Autodesk Fusion 360 part; units mm, degrees
(part 9 of 11)
  line L1964 (-0.0174, -45.4367) -> (0.0013, -45.4717)
  arc A128 (1.72, -193.2625) -> (1.3786, -193.1211) centre (1.52, -193.2625) ccw
  line L1965 (14.633, -219.988) -> (14.6722, -219.9945)
  arc A129 (1.72, -193.2625) -> (1.3786, -193.1211) centre (1.52, -193.2625) ccw
  line L1966 (14.6987, -220.198) -> (14.7482, -220.1997)
  line L1967 (6.02, -30.1995) -> (6.02, -32.839)
  line L1968 (3.3593, -195.4997) -> (1.72, -195.4997)
  line L1969 (3.7635, -37.4997) -> (7.1635, -34.0997)
  line L1970 (14.6722, -219.9945) -> (14.7117, -219.9984)
  line L1971 (6.02, -32.839) -> (3.3593, -35.4997)
  line L1972 (-0.0174, -45.4367) -> (0.0013, -45.4717)
  arc A130 (18.4614, -93.1211) -> (18.12, -93.2625) centre (18.32, -93.2625) ccw
  line L1973 (17.92, -144.6997) -> (17.92, -146.7368)
  line L1974 (19.9187, -145.2079) -> (19.92, -145.1682)
  line L1975 (15.42, -141.7997) -> (15.42, -143.439)
  arc A131 (18.4614, -93.1211) -> (18.12, -93.2625) centre (18.32, -93.2625) ccw
  line L1976 (17.92, -93.2625) -> (17.92, -95.2997)
  line L1977 (18.12, -93.2625) -> (18.12, -95.4997)
  line L1978 (16.4807, -144.4997) -> (18.12, -144.4997)
  line L1979 (16.4807, -144.4997) -> (18.12, -144.4997)
  line L1980 (18.12, -144.4997) -> (18.12, -146.7368)
  line L1981 (18.12, -93.2625) -> (18.12, -95.4997)
  line L1982 (19.7946, -94.4616) -> (19.7694, -94.4308)
  line L1983 (19.7422, -94.4019) -> (18.4614, -93.1211)
  line L1984 (16.5635, -144.6997) -> (17.92, -144.6997)
  arc A132 (18.12, -146.7368) -> (18.4614, -146.8782) centre (18.32, -146.7368) ccw
  arc A133 (18.6028, -92.9797) -> (17.92, -93.2625) centre (18.32, -93.2625) ccw
  line L1985 (19.7422, -94.4019) -> (18.4614, -93.1211)
  line L1986 (19.8859, -94.2627) -> (18.6028, -92.9797)
  arc A134 (18.12, -146.7368) -> (18.4614, -146.8782) centre (18.32, -146.7368) ccw
  line L1987 (14.7514, -139.9997) -> (18.42, -139.9997)
  line L1988 (15.42, -141.7997) -> (15.42, -143.439)
  arc A135 (17.92, -146.7368) -> (18.6028, -147.0197) centre (18.32, -146.7368) ccw
  line L1989 (18.42, -139.9997) -> (14.7514, -139.9997)
  line L1990 (19.92, -105.0997) -> (19.92, -94.8997)
  line L1991 (19.92, -105.0997) -> (19.92, -94.8997)
  line L1992 (19.7694, -94.4308) -> (19.7422, -94.4019)
  line L1993 (14.7482, -140.1997) -> (18.42, -140.1997)
  line L1994 (15.22, -141.9997) -> (15.22, -143.3562)
  line L1995 (19.7694, -94.4308) -> (19.7422, -94.4019)
  line L1996 (18.12, -144.4997) -> (18.12, -146.7368)
  line L1997 (20.12, -105.1009) -> (20.12, -94.8985)
  line L1998 (18.42, -139.9997) -> (14.7514, -139.9997)
  arc A136 (18.4614, -153.1211) -> (18.12, -153.2625) centre (18.32, -153.2625) ccw
  arc A137 (18.6028, -152.9797) -> (17.92, -153.2625) centre (18.32, -153.2625) ccw
  circle A138 centre (9.92, -149.9997) radius 2.1
  line L1999 (14.02, -152.7562) -> (14.02, -150.1167)
  line L2000 (16.1593, -157.2997) -> (18.12, -157.2997)
  line L2001 (17.92, -155.2997) -> (16.5635, -155.2997)
  line L2002 (18.12, -155.4997) -> (16.4807, -155.4997)
  arc A139 (18.4614, -153.1211) -> (18.12, -153.2625) centre (18.32, -153.2625) ccw
  line L2003 (18.12, -155.4997) -> (16.4807, -155.4997)
  line L2004 (10.127, -153.8997) -> (12.7593, -153.8997)
  line L2005 (13.82, -152.839) -> (13.82, -150.1995)
  line L2006 (5.82, -107.2432) -> (5.82, -109.8826)
  line L2007 (9.92, -153.6927) -> (10.127, -153.8997)
  line L2008 (13.903, -149.9997) -> (14.02, -149.8826)
  line L2009 (14.02, -150.1167) -> (13.903, -149.9997)
  circle A140 centre (9.92, -149.9997) radius 2.1
  line L2010 (9.92, -153.6927) -> (10.127, -153.8997)
  line L2011 (9.7959, -154.0997) -> (9.92, -153.9755)
  line L2012 (13.6201, -149.9997) -> (13.82, -149.7998)
  line L2013 (13.6201, -149.9997) -> (13.82, -149.7998)
  line L2014 (10.0441, -154.0997) -> (12.6765, -154.0997)
  line L2015 (14.3945, -80.1165) -> (14.4426, -80.1383)
  line L2016 (14.3222, -79.8219) -> (14.3512, -79.849)
  line L2017 (14.3819, -79.8742) -> (14.4142, -79.8974)
  line L2018 (16.5635, -124.6997) -> (17.92, -124.6997)
  line L2019 (14.483, -80.0623) -> (14.4479, -80.081)
  circle A141 centre (9.92, -129.9997) radius 2.1
  line L2020 (13.82, -130.1995) -> (13.6201, -129.9997)
  line L2021 (14.02, -132.7562) -> (14.02, -130.1167)
  line L2022 (14.4426, -79.861) -> (14.3945, -79.8828)
  line L2023 (14.3512, -79.849) -> (14.3819, -79.8742)
  line L2024 (14.3479, -79.9077) -> (14.303, -79.9356)
  line L2025 (14.4142, -80.102) -> (14.3819, -80.1251)
  line L2026 (14.483, -80.0623) -> (14.4479, -80.081)
  line L2027 (13.82, -130.1995) -> (13.6201, -129.9997)
  circle A142 centre (9.92, -129.9997) radius 2.1
  line L2028 (14.2601, -80.033) -> (14.303, -80.0637)
  line L2029 (14.5191, -80.0459) -> (14.483, -80.0623)
  line L2030 (14.3819, -79.8742) -> (14.4142, -79.8974)
  line L2031 (14.4142, -79.8974) -> (14.4479, -79.9183)
  line L2032 (14.3222, -79.8219) -> (14.3512, -79.849)
  line L2033 (14.7117, -79.9984) -> (14.7514, -79.9997)
  line L2034 (14.7117, -79.9984) -> (14.7514, -79.9997)
  line L2035 (1.72, -135.4997) -> (1.72, -133.2625)
  line L2036 (14.4426, -80.1383) -> (14.492, -80.1569)
  line L2037 (14.5425, -79.8271) -> (14.492, -79.8424)
  line L2038 (14.7514, -79.9997) -> (14.7117, -80.001)
  line L2039 (14.7482, -79.7997) -> (14.6987, -79.8013)
  line L2040 (6.02, -132.839) -> (3.3593, -135.4997)
  line L2041 (1.72, -135.4997) -> (1.72, -133.2625)
  line L2042 (14.5563, -80.0319) -> (14.5191, -80.0459)
  line L2043 (4.62, -136.6432) -> (7.1635, -134.0997)
  line L2044 (14.5563, -80.0319) -> (14.5191, -80.0459)
  line L2045 (3.2765, -135.2997) -> (1.92, -135.2997)
  line L2046 (14.5191, -79.9534) -> (14.5563, -79.9674)
  line L2047 (1.92, -135.2997) -> (1.92, -133.2625)
  line L2048 (14.6987, -80.198) -> (14.7482, -80.1997)
  arc A143 (1.72, -133.2625) -> (1.3786, -133.1211) centre (1.52, -133.2625) ccw
  line L2049 (14.3512, -80.1503) -> (14.3222, -80.1775)
  line L2050 (14.492, -80.1569) -> (14.5425, -80.1723)
  line L2051 (14.4479, -80.081) -> (14.4142, -80.102)
  line L2052 (14.5191, -79.9534) -> (14.5563, -79.9674)
  line L2053 (14.7514, -79.9997) -> (14.7117, -80.001)
  arc A144 (1.92, -133.2625) -> (1.2372, -132.9797) centre (1.52, -133.2625) ccw
  line L2054 (20.1184, -74.7783) -> (20.1132, -74.7258)
  line L2055 (19.8738, -74.5988) -> (19.8574, -74.5626)
  line L2056 (3.3593, -135.4997) -> (1.72, -135.4997)
  line L2057 (20.1046, -74.6736) -> (20.0926, -74.6222)
  line L2058 (6.02, -132.839) -> (3.3593, -135.4997)
  line L2059 (19.92, -74.8311) -> (19.9187, -74.7914)
  line L2060 (4.42, -136.5603) -> (7.0807, -133.8997)
  line L2061 (4.42, -136.5603) -> (7.0807, -133.8997)
  line L2062 (5.82, -132.7562) -> (3.2765, -135.2997)
  line L2063 (3.3593, -135.4997) -> (1.72, -135.4997)
  arc A145 (1.72, -133.2625) -> (1.3786, -133.1211) centre (1.52, -133.2625) ccw
  line L2064 (20.0926, -74.6222) -> (20.0773, -74.5717)
  line L2065 (20.1132, -74.7258) -> (20.1046, -74.6736)
  line L2066 (20.012, -74.4275) -> (19.9841, -74.3827)
  line L2067 (0.0978, -134.4019) -> (0.0706, -134.4308)
  line L2068 (19.8387, -74.5276) -> (19.8177, -74.4938)
  line L2069 (19.8387, -74.5276) -> (19.8177, -74.4938)
  line L2070 (19.9148, -74.7519) -> (19.9083, -74.7127)
  line L2071 (20.12, -78.4997) -> (20.12, -74.8278)
  line L2072 (-0.1969, -134.4741) -> (-0.2187, -134.5222)
  line L2073 (20.0773, -74.5717) -> (20.0587, -74.5222)
  line L2074 (19.9198, -74.2989) -> (19.8859, -74.2627)
  line L2075 (-0.2732, -134.7258) -> (-0.2786, -134.7804)
  line L2076 (19.8574, -74.5626) -> (19.8387, -74.5276)
  line L2077 (-0.172, -134.4275) -> (-0.1969, -134.4741)
  line L2078 (0.0454, -134.4616) -> (0.0223, -134.4938)
  line L2079 (20.12, -74.8278) -> (20.1184, -74.7783)
  line L2080 (-0.0174, -134.5626) -> (-0.0338, -134.5988)
  line L2081 (19.8993, -74.674) -> (19.8878, -74.636)
  line L2082 (-0.0478, -134.636) -> (-0.0593, -134.674)
  line L2083 (19.7694, -74.4308) -> (19.7422, -74.4019)
  line L2084 (19.8738, -74.5988) -> (19.8574, -74.5626)
  line L2085 (-0.0683, -134.7127) -> (-0.0748, -134.7519)
  line L2086 (-0.08, -54.8997) -> (-0.08, -65.0997)
  line L2087 (19.8177, -74.4938) -> (19.7946, -74.4616)
  line L2088 (0.0013, -134.5276) -> (-0.0174, -134.5626)
  line L2089 (-0.0593, -134.674) -> (-0.0683, -134.7127)
  line L2090 (-0.0683, -134.7127) -> (-0.0748, -134.7519)
  line L2091 (19.8878, -74.636) -> (19.8738, -74.5988)
  line L2092 (19.9187, -74.7914) -> (19.9148, -74.7519)
  line L2093 (-0.0787, -134.7914) -> (-0.08, -134.8997)
  line L2094 (-0.0338, -134.5988) -> (-0.0478, -134.636)
  line L2095 (-0.2187, -134.5222) -> (-0.2373, -134.5717)
  line L2096 (19.8177, -74.4938) -> (19.7946, -74.4616)
  line L2097 (20.0369, -74.4741) -> (20.012, -74.4275)
  line L2098 (19.8878, -74.636) -> (19.8738, -74.5988)
  line L2099 (-0.0748, -134.7519) -> (-0.0787, -134.7914)
  line L2100 (-0.0338, -134.5988) -> (-0.0478, -134.636)
  line L2101 (0.0978, -134.4019) -> (0.0706, -134.4308)
  line L2102 (19.9533, -74.3397) -> (19.9198, -74.2989)
  line L2103 (19.9841, -74.3827) -> (19.9533, -74.3397)
  line L2104 (19.7694, -74.4308) -> (19.7422, -74.4019)
  line L2105 (-0.0174, -134.5626) -> (-0.0338, -134.5988)
  line L2106 (19.9148, -74.7519) -> (19.9083, -74.7127)
  line L2107 (19.9187, -74.7914) -> (19.9148, -74.7519)
  line L2108 (-0.0478, -134.636) -> (-0.0593, -134.674)
  line L2109 (-0.1133, -134.3397) -> (-0.1441, -134.3827)
  line L2110 (19.8574, -74.5626) -> (19.8387, -74.5276)
  line L2111 (-0.2526, -134.6222) -> (-0.2646, -134.6736)
  line L2112 (19.9083, -74.7127) -> (19.8993, -74.674)
  line L2113 (0.0223, -134.4938) -> (0.0013, -134.5276)
  line L2114 (19.7946, -74.4616) -> (19.7694, -74.4308)
  line L2115 (-0.0798, -134.2989) -> (-0.1133, -134.3397)
  line L2116 (0.0706, -134.4308) -> (0.0454, -134.4616)
  line L2117 (1.92, -162.4997) -> (1.92, -157.4997)
  line L2118 (-0.0459, -134.2627) -> (-0.0798, -134.2989)
  line L2119 (17.92, -73.2625) -> (17.92, -75.2997)
  line L2120 (19.92, -74.8311) -> (19.9187, -74.7914)
  line L2121 (-0.2373, -134.5717) -> (-0.2526, -134.6222)
  line L2122 (-0.1441, -134.3827) -> (-0.172, -134.4275)
  line L2123 (-0.0787, -134.7914) -> (-0.08, -134.8997)
  line L2124 (20.0587, -74.5222) -> (20.0369, -74.4741)
  line L2125 (19.92, -78.4997) -> (19.92, -74.8311)
  line L2126 (0.0706, -134.4308) -> (0.0454, -134.4616)
  line L2127 (19.92, -78.4997) -> (19.92, -74.8311)
  line L2128 (-0.2646, -134.6736) -> (-0.2732, -134.7258)
  line L2129 (19.9083, -74.7127) -> (19.8993, -74.674)
  line L2130 (0.0013, -134.5276) -> (-0.0174, -134.5626)
  line L2131 (19.8993, -74.674) -> (19.8878, -74.636)
  line L2132 (19.7946, -74.4616) -> (19.7694, -74.4308)
  line L2133 (0.0223, -134.4938) -> (0.0013, -134.5276)
  line L2134 (-0.2786, -134.7804) -> (-0.28, -134.8985)
  line L2135 (18.12, -75.4997) -> (16.4807, -75.4997)
  line L2136 (5.937, -129.9997) -> (5.82, -130.1167)
  line L2137 (15.42, -76.5603) -> (15.42, -78.1997)
  arc A146 (18.4614, -73.1211) -> (18.12, -73.2625) centre (18.32, -73.2625) ccw
  line L2138 (1.3786, -133.1211) -> (0.0978, -134.4019)
  line L2139 (18.12, -73.2625) -> (18.12, -75.4997)
  line L2140 (1.2372, -132.9797) -> (-0.0459, -134.2627)
  line L2141 (19.8859, -74.2627) -> (18.6028, -72.9797)
  line L2142 (-0.0593, -134.674) -> (-0.0683, -134.7127)
  line L2143 (17.92, -75.2997) -> (16.5635, -75.2997)
  arc A147 (18.4614, -73.1211) -> (18.12, -73.2625) centre (18.32, -73.2625) ccw
  arc A148 (18.6028, -72.9797) -> (17.92, -73.2625) centre (18.32, -73.2625) ccw
  line L2144 (0.0454, -134.4616) -> (0.0223, -134.4938)
  line L2145 (15.22, -76.6432) -> (15.22, -77.9997)
  line L2146 (18.12, -73.2625) -> (18.12, -75.4997)
  line L2147 (-0.0748, -134.7519) -> (-0.0787, -134.7914)
  line L2148 (1.3786, -133.1211) -> (0.0978, -134.4019)
  line L2149 (15.42, -76.5603) -> (15.42, -78.1997)
  line L2150 (18.12, -75.4997) -> (16.4807, -75.4997)
  line L2151 (19.7422, -74.4019) -> (18.4614, -73.1211)
  arc A149 (1.3786, -126.8782) -> (1.72, -126.7368) centre (1.52, -126.7368) ccw
  line L2152 (19.7422, -74.4019) -> (18.4614, -73.1211)
  line L2153 (6.02, -127.1603) -> (6.02, -129.7998)
  line L2154 (19.92, -79.4997) -> (19.92, -78.4997)
  line L2155 (20.12, -79.4997) -> (20.12, -78.4997)
  line L2156 (5.82, -129.8826) -> (5.937, -129.9997)
  arc A150 (1.3786, -126.8782) -> (1.72, -126.7368) centre (1.52, -126.7368) ccw
  line L2157 (5.2837, -80.0319) -> (5.2457, -80.0203)
  line L2158 (19.9083, -114.7127) -> (19.8993, -114.674)
  line L2159 (19.8993, -114.674) -> (19.8878, -114.636)
  line L2160 (5.1678, -80.0049) -> (5.1283, -80.001)
  line L2161 (5.246, -79.8151) -> (5.1939, -79.8065)
  line L2162 (19.9148, -114.7519) -> (19.9083, -114.7127)
  line L2163 (18.12, -117.2997) -> (18.12, -122.6997)
  line L2164 (20.1046, -114.6736) -> (20.0926, -114.6222)
  line L2165 (19.8878, -114.636) -> (19.8738, -114.5988)
  line L2166 (5.1678, -79.9945) -> (5.207, -79.988)
  line L2167 (19.8878, -114.636) -> (19.8738, -114.5988)
  line L2168 (18.12, -122.6997) -> (16.1593, -122.6997)
  line L2169 (5.207, -80.0113) -> (5.1678, -80.0049)
  line L2170 (5.1678, -80.0049) -> (5.1283, -80.001)
  line L2171 (17.92, -122.4997) -> (16.0765, -122.4997)
  line L2172 (5.1283, -79.9984) -> (5.1678, -79.9945)
  line L2173 (19.9187, -114.7914) -> (19.9148, -114.7519)
  line L2174 (5.1413, -80.198) -> (5.1939, -80.1929)
  line L2175 (5.2457, -79.979) -> (5.2837, -79.9674)
  line L2176 (18.12, -117.2997) -> (18.12, -122.6997)
  line L2177 (5.2837, -80.0319) -> (5.2457, -80.0203)
  line L2178 (6.2199, -129.9997) -> (6.02, -130.1995)
  line L2179 (19.92, -65.0997) -> (19.92, -54.8997)
  arc A151 (1.2372, -127.0197) -> (1.92, -126.7368) centre (1.52, -126.7368) ccw
  line L2180 (12.9, -78.6825) -> (14.1831, -79.9656)
  line L2181 (10.0448, -74.0997) -> (12.6765, -74.0997)
  arc A152 (13.1828, -78.1997) -> (13.0414, -78.5411) centre (13.1828, -78.3997) ccw
  line L2182 (6.2199, -129.9997) -> (6.02, -130.1995)
  line L2183 (6.02, -129.7998) -> (6.2199, -129.9997)
  line L2184 (6.02, -129.7998) -> (6.2199, -129.9997)
  line L2185 (10.127, -73.8997) -> (12.7593, -73.8997)
  line L2186 (6.02, -127.1603) -> (6.02, -129.7998)
  line L2187 (9.7152, -73.8997) -> (9.92, -73.6949)
  arc A153 (13.1828, -77.9997) -> (12.9, -78.6825) centre (13.1828, -78.3997) ccw
  line L2188 (19.92, -79.4997) -> (19.92, -78.4997)
  line L2189 (9.7152, -73.8997) -> (9.92, -73.6949)
  line L2190 (10.127, -73.8997) -> (12.7593, -73.8997)
  line L2191 (9.7981, -74.0997) -> (9.9208, -73.977)
  line L2192 (9.92, -73.6949) -> (10.127, -73.8997)
  line L2193 (5.82, -127.2432) -> (5.82, -129.8826)
  line L2194 (1.72, -62.6997) -> (1.72, -57.2997)
  line L2195 (1.72, -124.4997) -> (3.3593, -124.4997)
  line L2196 (-0.2373, -125.4277) -> (-0.2187, -125.4771)
  line L2197 (9.92, -73.6949) -> (10.127, -73.8997)
  line L2198 (12.6765, -74.0997) -> (15.22, -76.6432)
  line L2199 (-0.2526, -125.3771) -> (-0.2373, -125.4277)
  arc A154 (13.1828, -78.1997) -> (13.0414, -78.5411) centre (13.1828, -78.3997) ccw
  line L2200 (-0.0748, -125.2474) -> (-0.0683, -125.2866)
  line L2201 (16.5635, -75.2997) -> (14.02, -72.7562)
  line L2202 (9.9208, -73.977) -> (10.0448, -74.0997)
  line L2203 (12.7593, -73.8997) -> (15.42, -76.5603)
  line L2204 (0.0013, -125.4717) -> (0.0223, -125.5055)
  line L2205 (13.0414, -78.5411) -> (14.3222, -79.8219)
  line L2206 (-0.28, -125.1009) -> (-0.2786, -125.2189)
  line L2207 (-0.1133, -125.6596) -> (-0.0798, -125.7004)
  line L2208 (-0.08, -125.0997) -> (-0.0787, -125.2079)
  line L2209 (15.42, -78.1997) -> (13.1828, -78.1997)
  line L2210 (0.0706, -125.5685) -> (0.0978, -125.5975)
  line L2211 (16.4807, -75.4997) -> (13.82, -72.839)
  line L2212 (14.1831, -79.9656) -> (14.2193, -79.9995)
  line L2213 (-0.0478, -125.3633) -> (-0.0338, -125.4005)
  line L2214 (15.42, -78.1997) -> (13.1828, -78.1997)
  line L2215 (12.7593, -73.8997) -> (15.42, -76.5603)
  line L2216 (-0.0593, -125.3253) -> (-0.0478, -125.3633)
  line L2217 (15.22, -77.9997) -> (13.1828, -77.9997)
  line L2218 (-0.0683, -125.2866) -> (-0.0593, -125.3253)
  line L2219 (13.0414, -78.5411) -> (14.3222, -79.8219)
  line L2220 (14.2193, -79.9999) -> (14.1831, -80.0337)
  line L2221 (-0.1441, -125.6166) -> (-0.1133, -125.6596)
  line L2222 (-0.0787, -125.2079) -> (-0.0748, -125.2474)
  line L2223 (-0.2786, -125.2189) -> (-0.2732, -125.2736)
  line L2224 (5.6569, -80.0337) -> (5.6207, -79.9999)
  line L2225 (-0.0338, -125.4005) -> (-0.0174, -125.4367)
  line L2226 (-0.2187, -125.4771) -> (-0.1969, -125.5252)
  line L2227 (-0.0787, -125.2079) -> (-0.0748, -125.2474)
  line L2228 (1.92, -124.6997) -> (3.2765, -124.6997)
  line L2229 (-0.0478, -125.3633) -> (-0.0338, -125.4005)
  line L2230 (5.6207, -79.9999) -> (5.5799, -79.9663)
  line L2231 (0.0454, -125.5378) -> (0.0706, -125.5685)
  line L2232 (-0.172, -125.5718) -> (-0.1441, -125.6166)
  line L2233 (-0.2646, -125.3257) -> (-0.2526, -125.3771)
  line L2234 (16.4807, -75.4997) -> (13.82, -72.839)
  line L2235 (5.537, -80.0637) -> (5.5799, -80.033)
  line L2236 (-0.08, -125.0997) -> (-0.0787, -125.2079)
  line L2237 (-0.0174, -125.4367) -> (0.0013, -125.4717)
  line L2238 (5.5799, -79.9663) -> (5.537, -79.9356)
  line L2239 (-0.0593, -125.3253) -> (-0.0478, -125.3633)
  line L2240 (-0.0174, -125.4367) -> (0.0013, -125.4717)
  line L2241 (0.0223, -125.5055) -> (0.0454, -125.5378)
  line L2242 (5.6207, -79.9995) -> (5.6569, -79.9656)
  line L2243 (0.0454, -125.5378) -> (0.0706, -125.5685)
  line L2244 (-0.1969, -125.5252) -> (-0.172, -125.5718)
  line L2245 (0.0013, -125.4717) -> (0.0223, -125.5055)
  line L2246 (-0.0748, -125.2474) -> (-0.0683, -125.2866)
  line L2247 (1.72, -124.4997) -> (3.3593, -124.4997)
  line L2248 (5.4581, -80.1251) -> (5.4258, -80.102)
  line L2249 (-0.2732, -125.2736) -> (-0.2646, -125.3257)
  line L2250 (0.0223, -125.5055) -> (0.0454, -125.5378)
  line L2251 (0.0706, -125.5685) -> (0.0978, -125.5975)
  line L2252 (-0.0798, -125.7004) -> (-0.0459, -125.7366)
  line L2253 (-0.0683, -125.2866) -> (-0.0593, -125.3253)
  line L2254 (5.3921, -80.081) -> (5.357, -80.0623)
  line L2255 (5.5799, -80.033) -> (5.6207, -79.9995)
  line L2256 (-0.0338, -125.4005) -> (-0.0174, -125.4367)
  line L2257 (5.4258, -79.8974) -> (5.4581, -79.8742)
  line L2258 (5.348, -80.1569) -> (5.3974, -80.1383)
  line L2259 (-0.0459, -125.7366) -> (1.2372, -127.0197)
  line L2260 (0.0978, -125.5975) -> (1.3786, -126.8782)
  line L2261 (5.4581, -79.8742) -> (5.4888, -79.849)
  line L2262 (5.357, -80.0623) -> (5.3209, -80.0459)
  line L2263 (6.02, -130.1995) -> (6.02, -132.839)
  line L2264 (1.72, -126.7368) -> (1.72, -124.4997)
  line L2265 (5.3974, -79.861) -> (5.348, -79.8424)
  line L2266 (5.4455, -79.8828) -> (5.3974, -79.861)
  line L2267 (1.92, -126.7368) -> (1.92, -124.6997)
  line L2268 (5.357, -79.9371) -> (5.3921, -79.9183)
  line L2269 (5.4455, -80.1165) -> (5.4921, -80.0916)
  line L2270 (0.0978, -125.5975) -> (1.3786, -126.8782)
  line L2271 (1.72, -126.7368) -> (1.72, -124.4997)
  line L2272 (5.4888, -80.1503) -> (5.4581, -80.1251)
  line L2273 (3.3593, -124.4997) -> (6.02, -127.1603)
  line L2274 (5.3921, -79.9183) -> (5.4258, -79.8974)
  line L2275 (3.3593, -124.4997) -> (6.02, -127.1603)
  line L2276 (3.2765, -124.6997) -> (5.82, -127.2432)
  line L2277 (5.82, -130.1167) -> (5.82, -132.7562)
  line L2278 (5.4258, -80.102) -> (5.3921, -80.081)
  line L2279 (5.3921, -79.9183) -> (5.4258, -79.8974)
  line L2280 (5.357, -79.9371) -> (5.3921, -79.9183)
  line L2281 (5.1939, -79.8065) -> (5.1413, -79.8013)
  line L2282 (7.0807, -133.8997) -> (9.7152, -133.8997)
  line L2283 (5.207, -79.988) -> (5.2457, -79.979)
  line L2284 (5.4258, -79.8974) -> (5.4581, -79.8742)
  line L2285 (5.3209, -79.9534) -> (5.357, -79.9371)
  line L2286 (7.1635, -134.0997) -> (9.7981, -134.0997)
  line L2287 (5.3921, -80.081) -> (5.357, -80.0623)
  line L2288 (5.4921, -79.9077) -> (5.4455, -79.8828)
  line L2289 (5.3209, -79.9534) -> (5.357, -79.9371)
  line L2290 (5.4888, -80.1503) -> (5.4581, -80.1251)
  line L2291 (7.0807, -133.8997) -> (9.7152, -133.8997)
  line L2292 (9.7959, -125.8997) -> (7.1635, -125.8997)
  line L2293 (5.357, -80.0623) -> (5.3209, -80.0459)
  line L2294 (9.713, -126.0997) -> (7.0807, -126.0997)
  line L2295 (5.4581, -80.1251) -> (5.4258, -80.102)
  line L2296 (9.713, -126.0997) -> (7.0807, -126.0997)
  line L2297 (6.02, -130.1995) -> (6.02, -132.839)
  line L2298 (5.3974, -80.1383) -> (5.4455, -80.1165)
  line L2299 (5.4581, -79.8742) -> (5.4888, -79.849)
  line L2300 (5.4258, -80.102) -> (5.3921, -80.081)
  line L2301 (5.1283, -79.9984) -> (5.1678, -79.9945)
  line L2302 (19.9187, -114.7914) -> (19.9148, -114.7519)
  line L2303 (5.2457, -80.0203) -> (5.207, -80.0113)
  line L2304 (0.0706, -154.4308) -> (0.0454, -154.4616)
  arc A155 (1.72, -153.2625) -> (1.3786, -153.1211) centre (1.52, -153.2625) ccw
  line L2305 (19.9083, -105.2866) -> (19.9148, -105.2474)
  line L2306 (6.2199, -149.9997) -> (6.02, -150.1995)
  line L2307 (-0.2526, -154.6222) -> (-0.2646, -154.6736)
  line L2308 (-0.0174, -154.5626) -> (-0.0338, -154.5988)
  line L2309 (0.0223, -154.4938) -> (0.0013, -154.5276)
  line L2310 (20.1186, -105.2189) -> (20.12, -105.1009)
  line L2311 (0.0223, -154.4938) -> (0.0013, -154.5276)
  line L2312 (-0.1441, -154.3827) -> (-0.172, -154.4275)
  line L2313 (0.0978, -154.4019) -> (0.0706, -154.4308)
  line L2314 (-0.172, -154.4275) -> (-0.1969, -154.4741)
  line L2315 (-0.0787, -154.7914) -> (-0.08, -154.8997)
  line L2316 (0.0706, -154.4308) -> (0.0454, -154.4616)
  arc A156 (1.92, -153.2625) -> (1.2372, -152.9797) centre (1.52, -153.2625) ccw
  line L2317 (-0.0478, -154.636) -> (-0.0593, -154.674)
  line L2318 (19.9841, -105.6166) -> (20.012, -105.5718)
  arc A157 (1.72, -153.2625) -> (1.3786, -153.1211) centre (1.52, -153.2625) ccw
  line L2319 (19.8177, -105.5055) -> (19.8387, -105.4717)
  line L2320 (20.1046, -105.3257) -> (20.1132, -105.2736)
  line L2321 (19.7946, -105.5378) -> (19.8177, -105.5055)
  line L2322 (19.8387, -105.4717) -> (19.8574, -105.4367)
  line L2323 (6.02, -152.839) -> (3.3593, -155.4997)
  line L2324 (19.9148, -105.2474) -> (19.9187, -105.2079)
  line L2325 (19.9187, -105.2079) -> (19.92, -105.0997)
  line L2326 (19.9148, -105.2474) -> (19.9187, -105.2079)
  line L2327 (19.9198, -105.7004) -> (19.9533, -105.6596)
  line L2328 (6.2199, -149.9997) -> (6.02, -150.1995)
  line L2329 (5.82, -149.8826) -> (5.937, -149.9997)
  line L2330 (20.0587, -105.4771) -> (20.0773, -105.4277)
  line L2331 (5.937, -149.9997) -> (5.82, -150.1167)
  line L2332 (6.02, -150.1995) -> (6.02, -152.839)
  line L2333 (6.02, -149.7998) -> (6.2199, -149.9997)
  line L2334 (5.82, -150.1167) -> (5.82, -152.7562)
  line L2335 (6.02, -150.1995) -> (6.02, -152.839)
  line L2336 (19.8574, -105.4367) -> (19.8738, -105.4005)
  line L2337 (6.02, -149.7998) -> (6.2199, -149.9997)
  line L2338 (19.8878, -105.3633) -> (19.8993, -105.3253)
  line L2339 (19.9533, -105.6596) -> (19.9841, -105.6166)
  line L2340 (1.72, -155.4997) -> (1.72, -153.2625)
  line L2341 (19.8878, -105.3633) -> (19.8993, -105.3253)
  line L2342 (20.012, -105.5718) -> (20.0369, -105.5252)
  line L2343 (20.1186, -94.7804) -> (20.1132, -94.7258)
  line L2344 (20.0369, -94.4741) -> (20.012, -94.4275)
  line L2345 (19.7694, -145.5685) -> (19.7946, -145.5378)
  line L2346 (19.8993, -145.3253) -> (19.9083, -145.2866)
  line L2347 (19.8878, -94.636) -> (19.8738, -94.5988)
  line L2348 (19.9148, -145.2474) -> (19.9187, -145.2079)
  line L2349 (20.0926, -94.6222) -> (20.0773, -94.5717)
  line L2350 (19.9841, -145.6166) -> (20.012, -145.5718)
  line L2351 (19.7946, -145.5378) -> (19.8177, -145.5055)
  line L2352 (20.12, -94.8985) -> (20.1186, -94.7804)
  line L2353 (19.8177, -94.4938) -> (19.7946, -94.4616)
  line L2354 (19.8738, -145.4005) -> (19.8878, -145.3633)
  line L2355 (20.1132, -145.2736) -> (20.1184, -145.221)
  line L2356 (20.0926, -145.3771) -> (20.1046, -145.3257)
  line L2357 (19.9198, -145.7004) -> (19.9533, -145.6596)
  line L2358 (19.8993, -94.674) -> (19.8878, -94.636)
  line L2359 (19.9198, -94.2989) -> (19.8859, -94.2627)
  line L2360 (19.8177, -145.5055) -> (19.8387, -145.4717)
  line L2361 (19.8574, -94.5626) -> (19.8387, -94.5276)
  line L2362 (20.012, -94.4275) -> (19.9841, -94.3827)
  line L2363 (20.1046, -145.3257) -> (20.1132, -145.2736)
  line L2364 (19.8859, -145.7366) -> (19.9198, -145.7004)
  line L2365 (17.92, -97.4997) -> (17.92, -102.4997)
  line L2366 (19.8387, -145.4717) -> (19.8574, -145.4367)
  line L2367 (19.7946, -145.5378) -> (19.8177, -145.5055)
  line L2368 (19.8177, -145.5055) -> (19.8387, -145.4717)
  line L2369 (18.6028, -107.0197) -> (19.8859, -105.7366)
  line L2370 (18.12, -97.2997) -> (18.12, -102.6997)
  line L2371 (18.12, -97.2997) -> (18.12, -102.6997)
  line L2372 (20.0773, -145.4277) -> (20.0926, -145.3771)
  line L2373 (19.8387, -145.4717) -> (19.8574, -145.4367)
  line L2374 (19.9148, -145.2474) -> (19.9187, -145.2079)
  line L2375 (19.9533, -145.6596) -> (19.9841, -145.6166)
  line L2376 (19.7422, -145.5975) -> (19.7694, -145.5685)
  line L2377 (20.0587, -145.4771) -> (20.0773, -145.4277)
  line L2378 (20.012, -145.5718) -> (20.0369, -145.5252)
  line L2379 (-0.2187, -154.5222) -> (-0.2373, -154.5717)
  line L2380 (0.0013, -154.5276) -> (-0.0174, -154.5626)
  line L2381 (-0.2646, -154.6736) -> (-0.2732, -154.7258)
  line L2382 (-0.0748, -154.7519) -> (-0.0787, -154.7914)
  line L2383 (-0.0593, -154.674) -> (-0.0683, -154.7127)
  line L2384 (-0.0338, -154.5988) -> (-0.0478, -154.636)
  line L2385 (-0.0787, -154.7914) -> (-0.08, -154.8997)
  line L2386 (-0.0174, -154.5626) -> (-0.0338, -154.5988)
  line L2387 (0.0013, -154.5276) -> (-0.0174, -154.5626)
  line L2388 (-0.0593, -154.674) -> (-0.0683, -154.7127)
  line L2389 (-0.0338, -154.5988) -> (-0.0478, -154.636)
  line L2390 (-0.0748, -154.7519) -> (-0.0787, -154.7914)
  line L2391 (-0.1133, -154.3397) -> (-0.1441, -154.3827)
  line L2392 (-0.0798, -154.2989) -> (-0.1133, -154.3397)
  line L2393 (0.0454, -154.4616) -> (0.0223, -154.4938)
  line L2394 (-0.1969, -154.4741) -> (-0.2187, -154.5222)
  line L2395 (-0.0459, -154.2627) -> (-0.0798, -154.2989)
  line L2396 (-0.2373, -154.5717) -> (-0.2526, -154.6222)
  line L2397 (-0.0478, -154.636) -> (-0.0593, -154.674)
  line L2398 (0.0978, -154.4019) -> (0.0706, -154.4308)
  line L2399 (-0.2786, -154.7804) -> (-0.28, -154.8985)
  line L2400 (-0.0683, -154.7127) -> (-0.0748, -154.7519)
  line L2401 (-0.2732, -154.7258) -> (-0.2786, -154.7804)
  line L2402 (-0.0683, -154.7127) -> (-0.0748, -154.7519)
  line L2403 (19.9148, -154.7519) -> (19.9083, -154.7127)
  line L2404 (20.0587, -154.5222) -> (20.0369, -154.4741)
  line L2405 (19.7694, -154.4308) -> (19.7422, -154.4019)
  line L2406 (20.1132, -154.7258) -> (20.1046, -154.6736)
  line L2407 (3.3593, -115.4997) -> (1.72, -115.4997)
  line L2408 (-0.2646, -114.6736) -> (-0.2732, -114.7258)
  line L2409 (-0.0593, -114.674) -> (-0.0683, -114.7127)
  line L2410 (-0.0478, -74.636) -> (-0.0593, -74.674)
  line L2411 (0.0706, -74.4308) -> (0.0454, -74.4616)
  line L2412 (-0.0478, -74.636) -> (-0.0593, -74.674)
  line L2413 (-0.0748, -74.7519) -> (-0.0787, -74.7914)
  line L2414 (3.6807, -122.6997) -> (1.72, -122.6997)
  line L2415 (0.0013, -114.5276) -> (-0.0174, -114.5626)
  line L2416 (-0.0593, -114.674) -> (-0.0683, -114.7127)
  line L2417 (-0.0174, -114.5626) -> (-0.0338, -114.5988)
  line L2418 (-0.0748, -74.7519) -> (-0.0787, -74.7914)
  line L2419 (1.72, -122.6997) -> (1.72, -117.2997)
  line L2420 (1.72, -122.6997) -> (1.72, -117.2997)
  line L2421 (-0.0338, -74.5988) -> (-0.0478, -74.636)
  line L2422 (0.0223, -74.4938) -> (0.0013, -74.5276)
  line L2423 (1.72, -117.2997) -> (3.6807, -117.2997)
  line L2424 (0.0454, -74.4616) -> (0.0223, -74.4938)
  line L2425 (-0.2786, -114.7804) -> (-0.28, -114.8985)
  line L2426 (-0.0683, -114.7127) -> (-0.0748, -114.7519)
  line L2427 (0.0223, -74.4938) -> (0.0013, -74.5276)
  line L2428 (-0.2373, -74.5717) -> (-0.2526, -74.6222)
  line L2429 (-0.0787, -114.7914) -> (-0.08, -114.8997)
  line L2430 (-0.2732, -114.7258) -> (-0.2786, -114.7804)
  line L2431 (-0.2646, -74.6736) -> (-0.2732, -74.7258)
  line L2432 (-0.0338, -114.5988) -> (-0.0478, -114.636)
  line L2433 (-0.28, -74.8985) -> (-0.28, -78.4997)
  line L2434 (-0.0787, -114.7914) -> (-0.08, -114.8997)
  line L2435 (-0.0683, -74.7127) -> (-0.0748, -74.7519)
  line L2436 (18.12, -157.2997) -> (18.12, -162.6997)
  line L2437 (0.0978, -74.4019) -> (0.0706, -74.4308)
  line L2438 (-0.0748, -114.7519) -> (-0.0787, -114.7914)
  line L2439 (-0.08, -74.8997) -> (-0.08, -78.4997)
  line L2440 (-0.2373, -114.5717) -> (-0.2526, -114.6222)
  line L2441 (-0.2187, -114.5222) -> (-0.2373, -114.5717)
  line L2442 (0.0013, -74.5276) -> (-0.0174, -74.5626)
  line L2443 (0.0013, -74.5276) -> (-0.0174, -74.5626)
  line L2444 (3.3593, -115.4997) -> (1.72, -115.4997)
  line L2445 (-0.1441, -74.3827) -> (-0.172, -74.4275)
  line L2446 (-0.2526, -74.6222) -> (-0.2646, -74.6736)
  line L2447 (1.92, -117.4997) -> (3.7635, -117.4997)
  line L2448 (-0.0683, -114.7127) -> (-0.0748, -114.7519)
  line L2449 (-0.1969, -74.4741) -> (-0.2187, -74.5222)
  line L2450 (1.72, -117.2997) -> (3.6807, -117.2997)
  line L2451 (0.0706, -74.4308) -> (0.0454, -74.4616)
  line L2452 (-0.0787, -74.7914) -> (-0.08, -74.8997)
  line L2453 (3.7635, -122.4997) -> (1.92, -122.4997)
  line L2454 (3.2765, -115.2997) -> (1.92, -115.2997)
  line L2455 (3.6807, -122.6997) -> (1.72, -122.6997)
  line L2456 (-0.0174, -74.5626) -> (-0.0338, -74.5988)
  line L2457 (0.0978, -74.4019) -> (0.0706, -74.4308)
  line L2458 (1.3786, -113.1211) -> (0.0978, -114.4019)
  line L2459 (1.2372, -72.9797) -> (-0.0459, -74.2627)
  line L2460 (-0.172, -74.4275) -> (-0.1969, -74.4741)
  arc A158 (1.92, -113.2625) -> (1.2372, -112.9797) centre (1.52, -113.2625) ccw
  line L2461 (1.3786, -73.1211) -> (0.0978, -74.4019)
  line L2462 (-0.0459, -74.2627) -> (-0.0798, -74.2989)
  line L2463 (-0.0338, -74.5988) -> (-0.0478, -74.636)
  line L2464 (-0.0174, -114.5626) -> (-0.0338, -114.5988)
  line L2465 (-0.0174, -74.5626) -> (-0.0338, -74.5988)
  arc A159 (1.72, -113.2625) -> (1.3786, -113.1211) centre (1.52, -113.2625) ccw
  line L2466 (-0.0593, -74.674) -> (-0.0683, -74.7127)
  line L2467 (-0.08, -74.8997) -> (-0.08, -78.4997)
  line L2468 (0.0013, -114.5276) -> (-0.0174, -114.5626)
  line L2469 (-0.2526, -114.6222) -> (-0.2646, -114.6736)
  line L2470 (-0.0787, -74.7914) -> (-0.08, -74.8997)
  line L2471 (-0.0748, -114.7519) -> (-0.0787, -114.7914)
  line L2472 (-0.2187, -74.5222) -> (-0.2373, -74.5717)
  line L2473 (-0.0338, -114.5988) -> (-0.0478, -114.636)
  line L2474 (-0.0683, -74.7127) -> (-0.0748, -74.7519)
  line L2475 (-0.1133, -74.3397) -> (-0.1441, -74.3827)
  line L2476 (0.0454, -74.4616) -> (0.0223, -74.4938)
  line L2477 (-0.0593, -74.674) -> (-0.0683, -74.7127)
  line L2478 (-0.172, -114.4275) -> (-0.1969, -114.4741)
  line L2479 (-0.0798, -114.2989) -> (-0.1133, -114.3397)
  arc A160 (1.72, -113.2625) -> (1.3786, -113.1211) centre (1.52, -113.2625) ccw
  line L2480 (0.0978, -114.4019) -> (0.0706, -114.4308)
  line L2481 (0.0706, -114.4308) -> (0.0454, -114.4616)
  line L2482 (5.6569, -79.9656) -> (6.94, -78.6825)
  line L2483 (1.3786, -73.1211) -> (0.0978, -74.4019)
  line L2484 (0.0706, -114.4308) -> (0.0454, -114.4616)
  line L2485 (-0.08, -78.4997) -> (-0.08, -79.4997)
  line L2486 (5.5178, -79.8219) -> (6.7986, -78.5411)
  line L2487 (0.0978, -114.4019) -> (0.0706, -114.4308)
  line L2488 (7.1635, -74.0997) -> (9.7981, -74.0997)
  line L2489 (-0.08, -78.4997) -> (-0.08, -79.4997)
  line L2490 (-0.28, -78.4997) -> (-0.28, -79.4997)
  line L2491 (-0.1441, -114.3827) -> (-0.172, -114.4275)
  line L2492 (7.0807, -73.8997) -> (9.7152, -73.8997)
  line L2493 (-0.0459, -114.2627) -> (-0.0798, -114.2989)
  line L2494 (1.2372, -112.9797) -> (-0.0459, -114.2627)
  line L2495 (5.5178, -79.8219) -> (6.7986, -78.5411)
  line L2496 (7.0807, -73.8997) -> (9.7152, -73.8997)
  line L2497 (1.3786, -113.1211) -> (0.0978, -114.4019)
  line L2498 (-0.1133, -114.3397) -> (-0.1441, -114.3827)
  line L2499 (0.0454, -114.4616) -> (0.0223, -114.4938)
  line L2500 (5.82, -112.7562) -> (3.2765, -115.2997)
  line L2501 (13.82, -70.1995) -> (13.6201, -69.9997)
  line L2502 (-0.1969, -114.4741) -> (-0.2187, -114.5222)
  line L2503 (6.02, -109.7998) -> (6.2199, -109.9997)
  line L2504 (0.0454, -114.4616) -> (0.0223, -114.4938)
  line L2505 (13.903, -69.9997) -> (14.02, -69.8826)
  line L2506 (6.02, -109.7998) -> (6.2199, -109.9997)
  line L2507 (6.02, -110.1995) -> (6.02, -112.839)
  line L2508 (14.02, -69.8826) -> (14.02, -67.2432)
  line L2509 (6.2199, -109.9997) -> (6.02, -110.1995)
  arc A161 (18.12, -66.7368) -> (18.4614, -66.8782) centre (18.32, -66.7368) ccw
  line L2510 (3.7635, -117.4997) -> (7.1635, -114.0997)
  line L2511 (13.82, -69.7998) -> (13.82, -67.1603)
  line L2512 (5.82, -110.1167) -> (5.82, -112.7562)
  line L2513 (5.82, -109.8826) -> (5.937, -109.9997)
  line L2514 (6.02, -110.1995) -> (6.02, -112.839)
  arc A162 (17.92, -66.7368) -> (18.6028, -67.0197) centre (18.32, -66.7368) ccw
  arc A163 (18.12, -66.7368) -> (18.4614, -66.8782) centre (18.32, -66.7368) ccw
  line L2515 (6.2199, -109.9997) -> (6.02, -110.1995)
  line L2516 (5.937, -109.9997) -> (5.82, -110.1167)
  line L2517 (14.02, -70.1167) -> (13.903, -69.9997)
  line L2518 (0.0223, -114.4938) -> (0.0013, -114.5276)
  line L2519 (7.0807, -113.8997) -> (9.713, -113.8997)
  line L2520 (16.0765, -122.4997) -> (12.6765, -125.8997)
  line L2521 (3.6807, -117.2997) -> (7.0807, -113.8997)
  line L2522 (7.0807, -113.8997) -> (9.713, -113.8997)
  line L2523 (6.02, -112.839) -> (3.3593, -115.4997)
  line L2524 (0.0223, -114.4938) -> (0.0013, -114.5276)
  line L2525 (13.82, -69.7998) -> (13.82, -67.1603)
  line L2526 (7.1635, -114.0997) -> (9.7959, -114.0997)
  line L2527 (6.02, -112.839) -> (3.3593, -115.4997)
  line L2528 (3.6807, -117.2997) -> (7.0807, -113.8997)
  line L2529 (13.82, -70.1995) -> (13.6201, -69.9997)
  line L2530 (1.92, -115.2997) -> (1.92, -113.2625)
  line L2531 (13.6201, -69.9997) -> (13.82, -69.7998)
  line L2532 (13.6201, -69.9997) -> (13.82, -69.7998)
  line L2533 (1.72, -115.4997) -> (1.72, -113.2625)
  line L2534 (1.72, -115.4997) -> (1.72, -113.2625)
  line L2535 (4.42, -138.1997) -> (4.42, -136.5603)
  line L2536 (19.8993, -65.3253) -> (19.9083, -65.2866)
  line L2537 (-0.08, -114.8997) -> (-0.08, -125.0997)
  line L2538 (7.1635, -125.8997) -> (3.7635, -122.4997)
  line L2539 (20.0773, -65.4277) -> (20.0926, -65.3771)
  line L2540 (19.92, -125.0997) -> (19.92, -114.8997)
  line L2541 (20.1132, -65.2736) -> (20.1186, -65.2189)
  line L2542 (19.92, -125.0997) -> (19.92, -114.8997)
  line L2543 (20.0926, -65.3771) -> (20.1046, -65.3257)
  line L2544 (16.1593, -122.6997) -> (12.7593, -126.0997)
  line L2545 (-0.08, -114.8997) -> (-0.08, -125.0997)
  line L2546 (20.12, -125.1009) -> (20.12, -114.8985)
  line L2547 (-0.28, -114.8985) -> (-0.28, -125.1009)
  line L2548 (7.0807, -126.0997) -> (3.6807, -122.6997)
  line L2549 (19.9187, -65.2079) -> (19.92, -65.0997)
  line L2550 (19.8177, -65.5055) -> (19.8387, -65.4717)
  line L2551 (20.1186, -65.2189) -> (20.12, -65.1009)
  line L2552 (19.8738, -65.4005) -> (19.8878, -65.3633)
  line L2553 (16.1593, -122.6997) -> (12.7593, -126.0997)
  line L2554 (-0.08, -134.8997) -> (-0.08, -138.4997)
  line L2555 (7.0807, -126.0997) -> (3.6807, -122.6997)
  line L2556 (19.9083, -65.2866) -> (19.9148, -65.2474)
  line L2557 (19.8387, -65.4717) -> (19.8574, -65.4367)
  line L2558 (19.9533, -65.6596) -> (19.9841, -65.6166)
  line L2559 (19.92, -138.4997) -> (19.92, -134.8311)
  line L2560 (19.7946, -65.5378) -> (19.8177, -65.5055)
  line L2561 (-0.28, -134.8985) -> (-0.28, -138.4997)
  line L2562 (15.42, -136.5603) -> (15.42, -138.1997)
  line L2563 (5.82, -192.7562) -> (3.2765, -195.2997)
  line L2564 (-0.0798, -205.7004) -> (-0.0459, -205.7366)
  line L2565 (5.4581, -219.8742) -> (5.4888, -219.849)
  line L2566 (6.2199, -189.9997) -> (6.02, -190.1995)
  line L2567 (0.0978, -165.5975) -> (1.3786, -166.8782)
  line L2568 (-0.2373, -165.4277) -> (-0.2187, -165.4771)
  line L2569 (-0.0174, -205.4367) -> (0.0013, -205.4717)
  line L2570 (5.3974, -220.1383) -> (5.4455, -220.1165)
  arc A164 (1.3786, -186.8782) -> (1.72, -186.7368) centre (1.52, -186.7368) ccw
  line L2571 (-0.1969, -205.5252) -> (-0.172, -205.5718)
  line L2572 (6.02, -189.7998) -> (6.2199, -189.9997)
  line L2573 (-0.1969, -165.5252) -> (-0.172, -165.5718)
  line L2574 (5.937, -189.9997) -> (5.82, -190.1167)
  line L2575 (-0.08, -205.0997) -> (-0.0787, -205.2079)
  line L2576 (-0.1441, -205.6166) -> (-0.1133, -205.6596)
  line L2577 (5.4921, -220.0916) -> (5.537, -220.0637)
  line L2578 (-0.0478, -205.3633) -> (-0.0338, -205.4005)
  line L2579 (-0.2786, -165.2189) -> (-0.2732, -165.2736)
  line L2580 (-0.2732, -165.2736) -> (-0.2646, -165.3257)
  line L2581 (5.0886, -219.9997) -> (5.1283, -219.9984)
  line L2582 (7.0807, -206.0997) -> (3.6807, -202.6997)
  line L2583 (-0.08, -194.8997) -> (-0.08, -205.0997)
  line L2584 (1.42, -220.1997) -> (5.0918, -220.1997)
  line L2585 (-0.2187, -205.4771) -> (-0.1969, -205.5252)
  line L2586 (0.0013, -205.4717) -> (0.0223, -205.5055)
  line L2587 (6.02, -167.1603) -> (6.02, -169.7998)
  line L2588 (5.1678, -219.9945) -> (5.207, -219.988)
  line L2589 (-0.0787, -205.2079) -> (-0.0748, -205.2474)
  line L2590 (1.42, -219.9997) -> (5.0886, -219.9997)
  line L2591 (5.82, -189.8826) -> (5.937, -189.9997)
  line L2592 (6.02, -187.1603) -> (6.02, -189.7998)
  line L2593 (5.4258, -219.8974) -> (5.4581, -219.8742)
  line L2594 (-0.28, -205.1009) -> (-0.2786, -205.2189)
  line L2595 (-0.1133, -205.6596) -> (-0.0798, -205.7004)
  line L2596 (1.42, -219.9997) -> (5.0886, -219.9997)
  line L2597 (5.82, -187.2432) -> (5.82, -189.8826)
  line L2598 (0.0013, -165.4717) -> (0.0223, -165.5055)
  line L2599 (0.0706, -165.5685) -> (0.0978, -165.5975)
  line L2600 (-0.0478, -165.3633) -> (-0.0338, -165.4005)
  line L2601 (5.2457, -219.979) -> (5.2837, -219.9674)
  arc A165 (-0.08, -219.4997) -> (0.42, -219.9997) centre (0.42, -219.4997) ccw
  line L2602 (-0.2646, -165.3257) -> (-0.2526, -165.3771)
  line L2603 (5.5799, -220.033) -> (5.6207, -219.9995)
  line L2604 (6.2199, -189.9997) -> (6.02, -190.1995)
  line L2605 (6.02, -189.7998) -> (6.2199, -189.9997)
  line L2606 (-0.0798, -165.7004) -> (-0.0459, -165.7366)
  line L2607 (6.02, -187.1603) -> (6.02, -189.7998)
  line L2608 (0.0013, -165.4717) -> (0.0223, -165.5055)
  line L2609 (5.4888, -219.849) -> (5.5178, -219.8219)
  line L2610 (0.42, -219.9997) -> (1.42, -219.9997)
  line L2611 (0.0013, -205.4717) -> (0.0223, -205.5055)
  line L2612 (0.42, -220.1997) -> (1.42, -220.1997)
  line L2613 (5.2837, -219.9674) -> (5.3209, -219.9534)
  line L2614 (5.537, -220.0637) -> (5.5799, -220.033)
  line L2615 (-0.0683, -205.2866) -> (-0.0593, -205.3253)
  arc A166 (-0.08, -219.4997) -> (0.42, -219.9997) centre (0.42, -219.4997) ccw
  arc A167 (1.3786, -186.8782) -> (1.72, -186.7368) centre (1.52, -186.7368) ccw
  line L2616 (-0.08, -194.8997) -> (-0.08, -205.0997)
  arc A168 (1.2372, -187.0197) -> (1.92, -186.7368) centre (1.52, -186.7368) ccw
  line L2617 (-0.08, -165.0997) -> (-0.0787, -165.2079)
  line L2618 (5.2975, -220.1723) -> (5.348, -220.1569)
  arc A169 (-0.28, -219.4997) -> (0.42, -220.1997) centre (0.42, -219.4997) ccw
  line L2619 (-0.08, -205.0997) -> (-0.0787, -205.2079)
  line L2620 (-0.0459, -165.7366) -> (1.2372, -167.0197)
  line L2621 (0.0454, -205.5378) -> (0.0706, -205.5685)
  line L2622 (0.0223, -205.5055) -> (0.0454, -205.5378)
  line L2623 (0.0978, -174.4019) -> (0.0706, -174.4308)
  line L2624 (-0.0787, -174.7914) -> (-0.08, -174.8997)
  line L2625 (1.72, -175.4997) -> (1.72, -173.2625)
  line L2626 (-0.28, -218.4997) -> (-0.28, -219.4997)
  line L2627 (5.246, -220.1843) -> (5.2975, -220.1723)
  line L2628 (5.2457, -219.979) -> (5.2837, -219.9674)
  line L2629 (3.3593, -175.4997) -> (1.72, -175.4997)
  line L2630 (0.0223, -205.5055) -> (0.0454, -205.5378)
  line L2631 (5.82, -167.2432) -> (5.82, -169.8826)
  line L2632 (-0.0338, -205.4005) -> (-0.0174, -205.4367)
  line L2633 (0.0706, -205.5685) -> (0.0978, -205.5975)
  line L2634 (3.2765, -175.2997) -> (1.92, -175.2997)
  line L2635 (5.3921, -219.9183) -> (5.4258, -219.8974)
  line L2636 (5.207, -219.988) -> (5.2457, -219.979)
  line L2637 (-0.0459, -205.7366) -> (1.2372, -207.0197)
  line L2638 (5.937, -169.9997) -> (5.82, -170.1167)
  line L2639 (5.1283, -219.9984) -> (5.1678, -219.9945)
  line L2640 (3.3593, -175.4997) -> (1.72, -175.4997)
  line L2641 (1.2372, -172.9797) -> (-0.0459, -174.2627)
  line L2642 (6.02, -172.839) -> (3.3593, -175.4997)
  line L2643 (0.42, -219.9997) -> (1.42, -219.9997)
  line L2644 (5.348, -220.1569) -> (5.3974, -220.1383)
  line L2645 (6.02, -170.1995) -> (6.02, -172.839)
  line L2646 (5.3209, -219.9534) -> (5.357, -219.9371)
  line L2647 (1.92, -175.2997) -> (1.92, -173.2625)
  arc A170 (1.72, -173.2625) -> (1.3786, -173.1211) centre (1.52, -173.2625) ccw
  line L2648 (6.02, -169.7998) -> (6.2199, -169.9997)
  line L2649 (6.02, -169.7998) -> (6.2199, -169.9997)
  line L2650 (5.82, -172.7562) -> (3.2765, -175.2997)
  line L2651 (-0.28, -194.8985) -> (-0.28, -205.1009)
  line L2652 (5.357, -219.9371) -> (5.3921, -219.9183)
  line L2653 (5.4258, -219.8974) -> (5.4581, -219.8742)
  line L2654 (5.4888, -219.849) -> (5.5178, -219.8219)
  line L2655 (6.02, -167.1603) -> (6.02, -169.7998)
  line L2656 (0.0978, -165.5975) -> (1.3786, -166.8782)
  line L2657 (-0.08, -218.4997) -> (-0.08, -219.4997)
  line L2658 (-0.2526, -205.3771) -> (-0.2373, -205.4277)
  line L2659 (5.4581, -219.8742) -> (5.4888, -219.849)
  line L2660 (5.1283, -219.9984) -> (5.1678, -219.9945)
  line L2661 (5.82, -169.8826) -> (5.937, -169.9997)
  line L2662 (0.0978, -174.4019) -> (0.0706, -174.4308)
  line L2663 (6.2199, -169.9997) -> (6.02, -170.1995)
  line L2664 (1.3786, -173.1211) -> (0.0978, -174.4019)
  line L2665 (1.3786, -173.1211) -> (0.0978, -174.4019)
  line L2666 (5.3209, -219.9534) -> (5.357, -219.9371)
  line L2667 (5.357, -219.9371) -> (5.3921, -219.9183)
  line L2668 (5.82, -170.1167) -> (5.82, -172.7562)
  line L2669 (6.02, -170.1995) -> (6.02, -172.839)
  line L2670 (6.2199, -169.9997) -> (6.02, -170.1995)
  line L2671 (-0.08, -218.4997) -> (-0.08, -219.4997)
  line L2672 (-0.0787, -205.2079) -> (-0.0748, -205.2474)
  line L2673 (-0.0593, -205.3253) -> (-0.0478, -205.3633)
  line L2674 (5.1413, -220.198) -> (5.1939, -220.1929)
  line L2675 (5.0886, -219.9997) -> (5.1283, -219.9984)
  line L2676 (5.6569, -219.9656) -> (6.94, -218.6825)
  line L2677 (1.72, -175.4997) -> (1.72, -173.2625)
  line L2678 (0.0454, -205.5378) -> (0.0706, -205.5685)
  line L2679 (5.1939, -220.1929) -> (5.246, -220.1843)
  arc A171 (1.92, -173.2625) -> (1.2372, -172.9797) centre (1.52, -173.2625) ccw
  line L2680 (6.02, -172.839) -> (3.3593, -175.4997)
  arc A172 (1.72, -173.2625) -> (1.3786, -173.1211) centre (1.52, -173.2625) ccw
  line L2681 (0.0223, -174.4938) -> (0.0013, -174.5276)
  line L2682 (-0.1133, -174.3397) -> (-0.1441, -174.3827)
  line L2683 (-0.2646, -174.6736) -> (-0.2732, -174.7258)
  line L2684 (0.0223, -174.4938) -> (0.0013, -174.5276)
  line L2685 (-0.0478, -174.636) -> (-0.0593, -174.674)
  line L2686 (-0.2526, -174.6222) -> (-0.2646, -174.6736)
  line L2687 (-0.0683, -174.7127) -> (-0.0748, -174.7519)
  line L2688 (-0.1969, -174.4741) -> (-0.2187, -174.5222)
  line L2689 (0.0013, -174.5276) -> (-0.0174, -174.5626)
  line L2690 (-0.2732, -174.7258) -> (-0.2786, -174.7804)
  line L2691 (-0.0459, -174.2627) -> (-0.0798, -174.2989)
  line L2692 (-0.0174, -174.5626) -> (-0.0338, -174.5988)
  line L2693 (-0.0478, -174.636) -> (-0.0593, -174.674)
  line L2694 (0.0454, -174.4616) -> (0.0223, -174.4938)
  line L2695 (-0.0748, -174.7519) -> (-0.0787, -174.7914)
  line L2696 (0.0454, -174.4616) -> (0.0223, -174.4938)
  line L2697 (-0.0593, -174.674) -> (-0.0683, -174.7127)
  line L2698 (-0.0748, -174.7519) -> (-0.0787, -174.7914)
  line L2699 (-0.0798, -174.2989) -> (-0.1133, -174.3397)
  line L2700 (-0.0338, -174.5988) -> (-0.0478, -174.636)
  line L2701 (-0.2187, -174.5222) -> (-0.2373, -174.5717)
  line L2702 (-0.0593, -174.674) -> (-0.0683, -174.7127)
  line L2703 (0.0706, -174.4308) -> (0.0454, -174.4616)
  line L2704 (-0.172, -174.4275) -> (-0.1969, -174.4741)
  line L2705 (-0.0174, -174.5626) -> (-0.0338, -174.5988)
  line L2706 (-0.2786, -174.7804) -> (-0.28, -174.8985)
  line L2707 (-0.1441, -174.3827) -> (-0.172, -174.4275)
  line L2708 (-0.2373, -174.5717) -> (-0.2526, -174.6222)
  line L2709 (-0.0787, -174.7914) -> (-0.08, -174.8997)
  line L2710 (-0.0338, -174.5988) -> (-0.0478, -174.636)
  line L2711 (0.0013, -174.5276) -> (-0.0174, -174.5626)
  line L2712 (-0.0683, -174.7127) -> (-0.0748, -174.7519)
  line L2713 (0.0706, -174.4308) -> (0.0454, -174.4616)
  line L2714 (0.0013, -65.4717) -> (0.0223, -65.5055)
  line L2715 (6.02, -27.1603) -> (6.02, -29.7998)
  line L2716 (-0.0787, -65.2079) -> (-0.0748, -65.2474)
  line L2717 (14.02, -29.8826) -> (14.02, -27.2432)
  line L2718 (-0.28, -65.1009) -> (-0.2786, -65.2189)
  line L2719 (20.012, -174.4275) -> (19.9841, -174.3827)
  line L2720 (14.3222, -80.1775) -> (13.0414, -81.4582)
  line L2721 (19.8387, -174.5276) -> (19.8177, -174.4938)
  line L2722 (-0.08, -65.0997) -> (-0.0787, -65.2079)
  line L2723 (-0.0748, -65.2474) -> (-0.0683, -65.2866)
  line L2724 (5.82, -27.2432) -> (5.82, -29.8826)
  line L2725 (19.92, -65.0997) -> (19.92, -54.8997)
  line L2726 (20.1186, -174.7804) -> (20.1132, -174.7258)
  line L2727 (19.8738, -174.5988) -> (19.8574, -174.5626)
  line L2728 (-0.0478, -65.3633) -> (-0.0338, -65.4005)
  line L2729 (-0.2646, -65.3257) -> (-0.2526, -65.3771)
  line L2730 (-0.28, -80.4997) -> (-0.28, -81.4997)
  line L2731 (13.82, -29.7998) -> (13.82, -27.1603)
  line L2732 (6.94, -81.3168) -> (5.6569, -80.0337)
  line L2733 (19.8574, -174.5626) -> (19.8387, -174.5276)
  line L2734 (20.12, -65.1009) -> (20.12, -54.8985)
  line L2735 (-0.08, -80.4997) -> (-0.08, -81.4997)
  line L2736 (20.1046, -174.6736) -> (20.0926, -174.6222)
  line L2737 (20.0926, -174.6222) -> (20.0773, -174.5717)
  line L2738 (1.72, -162.6997) -> (1.72, -157.2997)
  line L2739 (1.92, -62.4997) -> (1.92, -57.4997)
  line L2740 (19.9083, -174.7127) -> (19.8993, -174.674)
  line L2741 (14.1831, -80.0337) -> (12.9, -81.3168)
  line L2742 (6.02, -27.1603) -> (6.02, -29.7998)
  line L2743 (19.92, -81.4997) -> (19.92, -80.4997)
  line L2744 (13.82, -29.7998) -> (13.82, -27.1603)
  line L2745 (0.0454, -65.5378) -> (0.0706, -65.5685)
  line L2746 (20.0773, -174.5717) -> (20.0587, -174.5222)
  line L2747 (-0.0683, -65.2866) -> (-0.0593, -65.3253)
  line L2748 (19.9148, -174.7519) -> (19.9083, -174.7127)
  line L2749 (-0.0338, -65.4005) -> (-0.0174, -65.4367)
  line L2750 (-0.0787, -65.2079) -> (-0.0748, -65.2474)
  line L2751 (-0.1133, -65.6596) -> (-0.0798, -65.7004)
  line L2752 (20.1132, -174.7258) -> (20.1046, -174.6736)
  line L2753 (-0.2187, -65.4771) -> (-0.1969, -65.5252)
  line L2754 (20.12, -174.8985) -> (20.1186, -174.7804)
  line L2755 (19.92, -174.8997) -> (19.9187, -174.7914)
  line L2756 (14.3222, -80.1775) -> (13.0414, -81.4582)
  line L2757 (0.0223, -65.5055) -> (0.0454, -65.5378)
  line L2758 (-0.0798, -65.7004) -> (-0.0459, -65.7366)
  line L2759 (-0.08, -154.8997) -> (-0.08, -165.0997)
  line L2760 (19.8738, -174.5988) -> (19.8574, -174.5626)
  line L2761 (19.8177, -174.4938) -> (19.7946, -174.4616)
  line L2762 (6.02, -10.1995) -> (6.02, -12.839)
  arc A173 (18.4614, -173.1211) -> (18.12, -173.2625) centre (18.32, -173.2625) ccw
  line L2763 (20.0587, -174.5222) -> (20.0369, -174.4741)
  line L2764 (19.9083, -54.7127) -> (19.8993, -54.674)
  line L2765 (0.0223, -65.5055) -> (0.0454, -65.5378)
  line L2766 (-0.0748, -65.2474) -> (-0.0683, -65.2866)
  line L2767 (-0.08, -65.0997) -> (-0.0787, -65.2079)
  line L2768 (19.8993, -174.674) -> (19.8878, -174.636)
  line L2769 (16.1593, -42.6997) -> (12.7593, -46.0997)
  line L2770 (19.92, -81.4997) -> (19.92, -80.4997)
  line L2771 (6.7986, -81.4582) -> (5.5178, -80.1775)
  line L2772 (-0.0478, -65.3633) -> (-0.0338, -65.4005)
  line L2773 (-0.0683, -65.2866) -> (-0.0593, -65.3253)
  line L2774 (1.72, -162.6997) -> (1.72, -157.2997)
  line L2775 (-0.2786, -65.2189) -> (-0.2732, -65.2736)
  line L2776 (16.0765, -42.4997) -> (12.6765, -45.8997)
  line L2777 (19.92, -174.8997) -> (19.9187, -174.7914)
  line L2778 (6.02, -10.1995) -> (6.02, -12.839)
  line L2779 (0.0013, -65.4717) -> (0.0223, -65.5055)
  line L2780 (19.8878, -174.636) -> (19.8738, -174.5988)
  line L2781 (-0.1969, -65.5252) -> (-0.172, -65.5718)
  line L2782 (-0.28, -154.8985) -> (-0.28, -165.1009)
  line L2783 (-0.08, -34.8997) -> (-0.08, -45.0997)
  line L2784 (-0.0174, -65.4367) -> (0.0013, -65.4717)
  line L2785 (19.9198, -174.2989) -> (19.8859, -174.2627)
  line L2786 (5.82, -10.1167) -> (5.82, -12.7562)
  line L2787 (19.7946, -174.4616) -> (19.7694, -174.4308)
  line L2788 (14.02, -12.7562) -> (14.02, -10.1167)
  line L2789 (6.7986, -81.4582) -> (5.5178, -80.1775)
  line L2790 (19.9198, -54.2989) -> (19.8859, -54.2627)
  line L2791 (-0.0593, -65.3253) -> (-0.0478, -65.3633)
  line L2792 (13.82, -12.839) -> (13.82, -10.1995)
  line L2793 (20.12, -81.4997) -> (20.12, -80.4997)
  line L2794 (19.9841, -174.3827) -> (19.9533, -174.3397)
  line L2795 (-0.172, -65.5718) -> (-0.1441, -65.6166)
  line L2796 (-0.2732, -65.2736) -> (-0.2646, -65.3257)
  line L2797 (19.9841, -54.3827) -> (19.9533, -54.3397)
  line L2798 (19.9187, -174.7914) -> (19.9148, -174.7519)
  line L2799 (19.92, -45.0997) -> (19.92, -34.8997)
  line L2800 (13.82, -12.839) -> (13.82, -10.1995)
  line L2801 (-0.28, -34.8985) -> (-0.28, -45.1009)